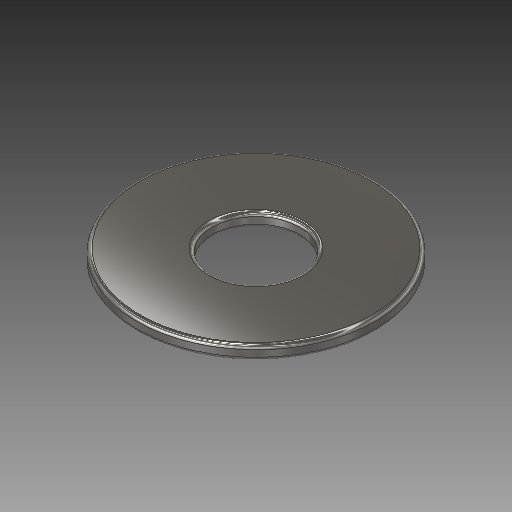
# Autodesk Inventor part: paris_washer
Saved by Autodesk Inventor 2019.3 (Build 233278000, 278)
## iProperties
Created: 2017-04-02
Part Number: paris_washer
Material: Типовые
Document SubType Name: Modeling
Designer: Nikita
Density: 1 g/cm^3
Appearance: Сталь — полированная
Mass: 0.682412 g
Surface Area: 10.4909 cm^2
Volume: 0.682412 cm^3
Author: Nikita
Autodesk Inventor part; units mm, degrees
ref_plane "YZ Plane" through (0, 0, 0) normal (1, 0, 0) x (0, 1, 0)
ref_plane "XZ Plane" through (0, 0, 0) normal (0, 1, 0) x (-1, 0, 0)
ref_plane "XY Plane" through (0, 0, 0) normal (0, 0, 1) x (1, 0, 0)
sketch "Эскиз1" plane through (0, 0, 0) normal (0, 0, 1) x (1, 0, 0)
  line L0 (4.75, 0) -> (13, 0)
  line L1 (13, 0) -> (13, 1.5)
  line L2 (13, 1.5) -> (4.75, 1.5)
  line L3 (0, 1.5) -> (0, 0)
  line L4 (4.75, 1.5) -> (4.75, 0)
  dimension "d0" = 26
  dimension "d3" = 1.5
  dimension "d7" = 9.5
  constraints: 10 end point, 3 perpendicular, 1 horizontal, 1 parallel, 1 point on line
  measures "d0" diameter of L1 L3
  measures "d3" distance between parallel lines of L0 L2
  measures "d7" diameter of L4 L3
revolve "Вращение1" add sketch "Эскиз1" angle 360 about axis through (0, 1.5, 0) along (0, -1, 0)
fillet "Сопряжение3" radius 0.4 4 edges at (-13, 0, 0) (-13, 1.5, 0) (-4.75, 0, 0) (-4.75, 1.5, 0)
equation "\"d3\" = d2"
equation "\"d2\" = 1.5"
